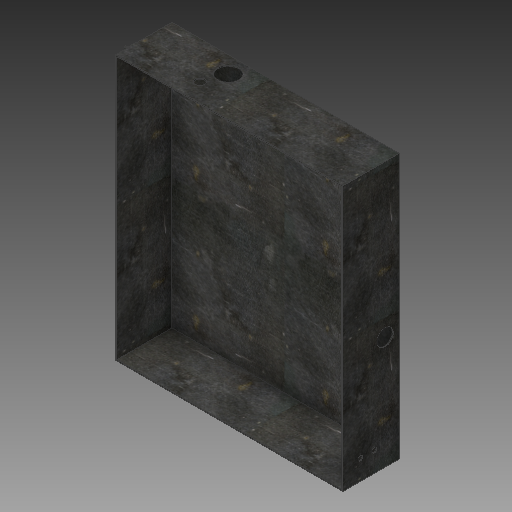
# Autodesk Inventor part: case
Saved by Autodesk Inventor 2018 (Build 220112000, 112)
## iProperties
Created: 2018-08-03
Part Number: case
Material: Steel
Document SubType Name: Modeling
Designer: Cole Tucker
Density: 7.85 g/cm^3
Appearance: Plate
Mass: 2647.98 g
Surface Area: 4223.8 cm^2
Volume: 337.322 cm^3
Author: Cole Tucker
Autodesk Inventor part; units mm, degrees
ref_plane "YZ Plane" through (0, 0, 0) normal (1, 0, 0) x (0, 1, 0)
ref_plane "XZ Plane" through (0, 0, 0) normal (0, 1, 0) x (-1, 0, 0)
ref_plane "XY Plane" through (0, 0, 0) normal (0, 0, 1) x (1, 0, 0)
sketch "Sketch1" plane through (0, 0, 0) normal (0, 0, 1) x (1, 0, 0)
  line L0 (0, 0) -> (307.975, 0)
  line L1 (307.975, 0) -> (307.975, 358.775)
  line L2 (307.975, 358.775) -> (0, 358.775)
  line L3 (0, 358.775) -> (0, 0)
  dimension "d0" = 307.975
  dimension "d1" = 358.775
  constraints: 8 end point, 2 parallel, 1 horizontal, 1 perpendicular
  measures "d0" distance of L2.end L1.end
  measures "d1" distance of L2.end L0.start
extrude "Extrusion1" add sketch "Sketch1" along normal blind 76.2
shell "Shell1" thickness 1.5875 removed faces 1 at (205.3167, 119.5917, 76.2)
sketch "Sketch2" plane through (0, 358.775, 0) normal (0, 1, 0) x (1, 0, 0)
  line L0 (0, -76.2) -> (0, -60.325) construction
  line L1 (0, -60.325) -> (-3.175, -60.325) construction
  arc A0 (-2.3813, -58.7375) -> (-0.7938, -60.325) centre (-2.3813, -60.325) ccw
  line L2 (0, -60.325) -> (-0.7938, -60.325)
  line L3 (-0.7938, -58.7375) -> (-0.7938, -47.625)
  line L4 (-0.7938, -47.625) -> (0, -47.625)
  line L5 (0, -47.625) -> (0, -60.325)
  line L6 (-2.3813, -58.7375) -> (-0.7938, -58.7375)
  point P0 (0, 0)
  dimension "d10" = 15.875
  dimension "d11" = 3.175
  dimension "d12" = 3.175
  dimension "d13" = 12.7
  constraints: 14 end point, 3 perpendicular, 2 parallel, 2 point on circle, 1 centre point, 1 horizontal, 1 point on line, 1 tangent
  measures "d10" distance of L0.start L0.end
  measures "d11" distance of L0.end L1.end
  measures "d12" diameter of A0
  measures "d13" distance of L2.end L3.end
extrude "Extrusion2" add sketch "Sketch2" against normal up to surface (358.775 mm away)
sketch "Sketch3" plane through (307.975, 0, 0) normal (1, 0, 0) x (0, 0, -1)
  line L0 (0, 358.775) -> (0, 0) construction
  line L1 (0, 0) -> (-19.05, 0) construction
  line L2 (-19.05, 0) -> (-19.05, 152.4) construction
  line L3 (-19.05, 152.4) -> (0, 152.4) construction
  line L4 (0, 152.4) -> (0, 0) construction
  dimension "d14" = 19.05
  dimension "d15" = 152.4
  constraints: 8 end point, 2 parallel, 1 coincident, 1 horizontal, 1 perpendicular
  measures "d14" distance of L2.end L3.end
  measures "d15" distance of L1.end L2.end
hole "Hole1" at (307.975, 152.4, 19.05) direction (-1, 0, 0) diameter 22.225 depth 25.4 tip angle 118
sketch "Sketch4" plane through (307.975, 0, 0) normal (1, 0, 0) x (0, 0, -1)
  line L0 (-1.5875, 357.1875) -> (-1.5875, 1.5875) construction
  line L1 (-1.5875, 1.5875) -> (-1.5875, 26.9875) construction
  line L2 (-1.5875, 26.9875) -> (-33.3375, 26.9875) construction
  line L3 (-1.5875, 26.9875) -> (-52.3875, 26.9875) construction
  point P0 (0, 0)
  dimension "d23" = 25.4
  dimension "d24" = 31.75
  dimension "d25" = 50.8
  constraints: 6 end point, 2 coincident, 2 point on line, 1 perpendicular
  measures "d23" distance of L0.end L1.end
  measures "d24" distance of L1.end L2.end
  measures "d25" distance of L1.end L3.end
hole "Hole2" at (307.975, 26.9875, 52.3875) at (307.975, 26.9875, 33.3375) direction (-1, 0, 0) diameter 6.35 depth 25.4 tip angle 118
sketch "Sketch5" plane through (0, 358.775, 0) normal (0, 1, 0) x (1, 0, 0)
  line L0 (0, 0) -> (307.975, 0) projected
  line L1 (0, 0) -> (98.425, 0)
  line L2 (98.425, 0) -> (98.425, -22.225)
  dimension "d33" = 98.425
  dimension "d34" = 22.225
  constraints: 4 end point, 1 coincident, 1 perpendicular, 1 point on line
  measures "d33" distance of L0.start L1.end
  measures "d34" distance of L1.end L2.end
hole "Hole3" at (98.425, 358.775, 22.225) direction (0, -1, 0) diameter 28.575 depth 25.4 tip angle 118
sketch "Sketch6" plane through (0, 358.775, 0) normal (0, 1, 0) x (1, 0, 0)
  line L0 (0, -76.2) -> (307.975, -76.2) construction
  line L1 (0, -76.2) -> (88.9, -76.2) construction
  line L2 (88.9, -76.2) -> (88.9, -50.8) construction
  line L3 (88.9, -50.8) -> (0, -50.8) construction
  line L4 (0, -50.8) -> (0, -76.2) construction
  point P0 (0, 0)
  dimension "d42" = 88.9
  dimension "d43" = 25.4
  constraints: 8 end point, 2 parallel, 1 coincident, 1 horizontal, 1 perpendicular
  measures "d42" distance of L3.end L2.end
  measures "d43" distance of L2.end L1.end
hole "Hole4" at (88.9, 358.775, 50.8) direction (0, -1, 0) diameter 12.7 depth 25.4 tip angle 118
body "Solid1"
